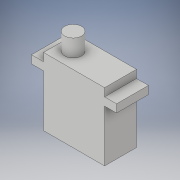
# Autodesk Inventor part: sg90_servo
Saved by Autodesk Inventor 2018 (Build 220112000, 112)
## iProperties
Created: 2018-03-22
Part Number: sg90_servo
Material: Generic
Document SubType Name: Modeling
Designer: scwu
Density: 1 g/cm^3
Appearance: Default
Author: scwu
Autodesk Inventor part; units mm, degrees
ref_plane "YZ Plane" through (0, 0, 0) normal (1, 0, 0) x (0, 1, 0)
ref_plane "XZ Plane" through (0, 0, 0) normal (0, 1, 0) x (-1, 0, 0)
ref_plane "XY Plane" through (0, 0, 0) normal (0, 0, 1) x (1, 0, 0)
sketch "Sketch1" plane through (0, 0, 0) normal (0, 1, 0) x (-1, 0, 0)
  line L0 (11.5, -6) -> (-11.5, -6)
  line L1 (-11.5, -6) -> (-11.5, 6)
  line L2 (-11.5, 6) -> (11.5, 6)
  line L3 (11.5, 6) -> (11.5, -6)
  line L4 (11.5, -6) -> (-11.5, 6) construction
  line L5 (-11.5, -6) -> (11.5, 6) construction
  point P0 (0, 0)
  dimension "d0" = 23
  dimension "d1" = 12
  constraints: 12 end point, 2 midpoint, 2 parallel, 1 horizontal, 1 perpendicular
  measures "d0" distance of L1.end L2.end
  measures "d1" distance of L0.end L1.end
extrude "Extrusion1" add sketch "Sketch1" along normal blind 19.5
sketch "Sketch2" plane through (0, 19.5, 0) normal (0, 1, 0) x (1, 0, 0)
  line L0 (16, -6) -> (-16, -6)
  line L1 (-16, -6) -> (-16, 6)
  line L2 (-16, 6) -> (16, 6)
  line L3 (16, 6) -> (16, -6)
  line L4 (16, -6) -> (-16, 6) construction
  line L5 (-16, -6) -> (16, 6) construction
  point P0 (0, 0)
  dimension "d4" = 32
  dimension "d5" = 12
  constraints: 12 end point, 2 midpoint, 2 parallel, 1 horizontal, 1 perpendicular
  measures "d4" distance of L1.end L2.end
  measures "d5" distance of L0.end L1.end
extrude "Extrusion2" add sketch "Sketch2" along normal blind 3
sketch "Sketch3" plane through (0, 22.5, 0) normal (0, 1, 0) x (1, 0, 0)
  line L0 (11.5, 6) -> (16, 6) projected
  line L1 (-11.5, -6) -> (11.5, -6)
  line L2 (11.5, -6) -> (11.5, 6)
  line L3 (11.5, 6) -> (-11.5, 6)
  line L4 (-11.5, 6) -> (-11.5, -6)
  line L5 (-11.5, -6) -> (11.5, 6) construction
  line L6 (11.5, -6) -> (-11.5, 6) construction
  point P0 (0, 0)
  constraints: 12 end point, 2 midpoint, 2 parallel, 1 horizontal, 1 perpendicular
extrude "Extrusion3" add sketch "Sketch3" along normal blind 3
sketch "Sketch4" plane through (0, 25.5, 0) normal (0, 1, 0) x (1, 0, 0)
  circle A0 centre (-6.35, 0) radius 3.175
  point P0 (0, 0)
  dimension "d10" = 6.35
  constraints: 1 centre point
  measures "d10" diameter of A0
extrude "Extrusion4" add sketch "Sketch4" along normal blind 6.5
body "Solid1"
